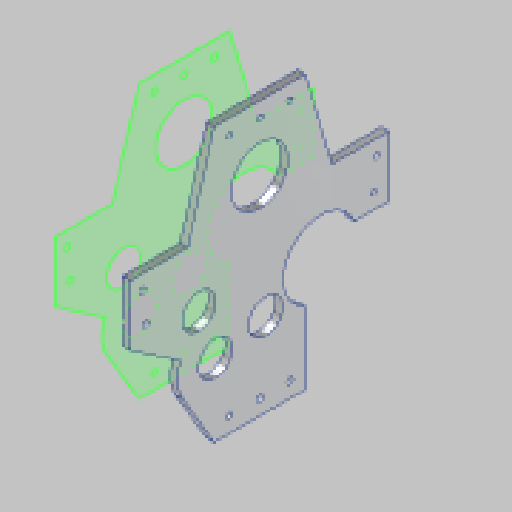
# Autodesk Inventor part: EL2-CGB-003
Saved by Autodesk Inventor 2023.5 (Build 275446000, 446)
## iProperties
Created: 2025-01-19
Part Number: EL2-CGB-003
Material: Aluminum 6061
Document SubType Name: Modeling
Designer: mavericks
Density: 2.7 g/cm^3
Appearance: Aluminum - Flat
Author: mavericks
Autodesk Inventor part; units mm, degrees
ref_plane "YZ Plane" through (0, 0, 0) normal (1, 0, 0) x (0, 1, 0)
ref_plane "XZ Plane" through (0, 0, 0) normal (0, 1, 0) x (-1, 0, 0)
ref_plane "XY Plane" through (0, 0, 0) normal (0, 0, 1) x (1, 0, 0)
sketch "Sketch1" plane through (0, 0, 0) normal (1, 0, 0) x (0, 1, 0)
  line L0 (127, 107.95) -> (-127, 107.95) construction
  line L1 (-127, 107.95) -> (-127, 82.55) construction
  line L2 (-127, 82.55) -> (127, 82.55) construction
  line L3 (127, 82.55) -> (127, 107.95) construction
  line L4 (-44.45, 128.7526) -> (-69.85, 128.7526) construction
  line L5 (-69.85, 128.7526) -> (-69.85, 79.4258) construction
  line L6 (-69.85, 79.4258) -> (-44.45, 79.4258) construction
  line L7 (-44.45, 79.4258) -> (-44.45, 128.7526) construction
  line L8 (69.85, 128.7526) -> (44.45, 128.7526) construction
  line L9 (44.45, 128.7526) -> (44.45, 79.4258) construction
  line L10 (44.45, 79.4258) -> (69.85, 79.4258) construction
  line L11 (69.85, 79.4258) -> (69.85, 128.7526) construction
  line L12 (44.45, 104.0892) -> (-44.45, 104.0892) construction
  line L13 (0, 0) -> (-27.2932, 0) construction
  line L14 (127, -107.95) -> (-127, -107.95) construction
  line L15 (-127, -107.95) -> (-127, -82.55) construction
  line L16 (-127, -82.55) -> (127, -82.55) construction
  line L17 (127, -82.55) -> (127, -107.95) construction
  line L18 (-44.45, -128.7526) -> (-69.85, -128.7526) construction
  line L19 (-69.85, -128.7526) -> (-69.85, -79.4258) construction
  line L20 (-69.85, -79.4258) -> (-44.45, -79.4258) construction
  line L21 (-44.45, -79.4258) -> (-44.45, -128.7526) construction
  line L22 (69.85, -128.7526) -> (44.45, -128.7526) construction
  line L23 (44.45, -128.7526) -> (44.45, -79.4258) construction
  line L24 (44.45, -79.4258) -> (69.85, -79.4258) construction
  line L25 (69.85, -79.4258) -> (69.85, -128.7526) construction
  line L26 (44.45, -104.0892) -> (-44.45, -104.0892) construction
  line L27 (127, 82.55) -> (101.6, 82.55) construction
  line L28 (101.6, 82.55) -> (101.6, -82.55) construction
  line L29 (101.6, -82.55) -> (127, -82.55) construction
  line L30 (127, -82.55) -> (127, 82.55) construction
  line L31 (-127, 82.55) -> (-101.6, 82.55) construction
  line L32 (-101.6, 82.55) -> (-101.6, -82.55) construction
  line L33 (-101.6, -82.55) -> (-127, -82.55) construction
  line L34 (-127, -82.55) -> (-127, 82.55) construction
  point P0 (0, 82.55)
  point P1 (0, 104.0892)
  point P2 (0, -82.55)
  point P3 (0, -104.0892)
  dimension "d0" = 254
  dimension "d1" = 25.4
  dimension "d2" = 82.55
  dimension "d3" = 25.4
  dimension "d4" = 49.3268
  dimension "d6" = 88.9
  dimension "d7" = 3.1242
  dimension "d8" = 25.4
  dimension "d9" = 25.4
  constraints: 70 end point, 16 symmetric about line, 12 parallel, 7 horizontal, 5 perpendicular, 4 midpoint, 2 vertical alignment, 1 horizontal alignment, 1 point on line
  measures "d0" distance of L2.end L1.end
  measures "d1" distance of L1.end L0.end
  measures "d2" vertical distance of L13.start L2.end
  measures "d3" distance of L6.end L5.end
  measures "d4" distance of L5.end L4.end
  measures "d6" distance of L4.start L8.end
  measures "d7" distance from line of L2 L6.end
  measures "d8" distance between parallel lines of L28 L30
  measures "d9" distance between parallel lines of L34 L32
sketch "Sketch2" plane through (0, 0, 0) normal (1, 0, 0) x (0, 1, 0)
  line L0 (-127, 107.95) -> (-127, 82.55) construction
  line L1 (44.45, 104.0892) -> (-44.45, 104.0892) construction
  line L2 (-127, 82.55) -> (127, 82.55) construction
  line L3 (127, 107.95) -> (-127, 107.95) construction
  line L4 (44.45, 79.4258) -> (69.85, 79.4258) construction
  line L5 (127, 82.55) -> (127, 107.95) construction
  line L6 (-69.85, 79.4258) -> (-44.45, 79.4258) construction
  line L7 (-44.45, 79.4258) -> (-44.45, 128.7526) construction
  line L8 (-69.85, 128.7526) -> (-69.85, 79.4258) construction
  line L9 (-44.45, 128.7526) -> (-69.85, 128.7526) construction
  line L10 (101.6, 82.55) -> (101.6, -82.55) construction
  line L11 (127, -82.55) -> (127, 82.55) construction
  line L12 (-127, -82.55) -> (127, -82.55) construction
  line L13 (127, -107.95) -> (-127, -107.95) construction
  line L14 (44.45, -104.0892) -> (-44.45, -104.0892) construction
  line L15 (-127, 82.55) -> (-101.6, 82.55) construction
  line L16 (-101.6, 82.55) -> (-101.6, -82.55) construction
  line L17 (-127, -82.55) -> (-127, 82.55) construction
  line L18 (-69.85, -79.4258) -> (-44.45, -79.4258) construction
  line L19 (-101.6, -82.55) -> (-127, -82.55) construction
  line L20 (-44.45, -79.4258) -> (-44.45, -128.7526) construction
  line L21 (-44.45, -128.7526) -> (-69.85, -128.7526) construction
  line L22 (-69.85, -128.7526) -> (-69.85, -79.4258) construction
  line L23 (-127, -107.95) -> (-127, -82.55) construction
  line L24 (44.45, -79.4258) -> (69.85, -79.4258) construction
  line L25 (44.45, -128.7526) -> (44.45, -79.4258) construction
  line L26 (101.6, -82.55) -> (127, -82.55) construction
  line L27 (69.85, -128.7526) -> (44.45, -128.7526) construction
  line L28 (69.85, -79.4258) -> (69.85, -128.7526) construction
  line L29 (127, -82.55) -> (127, -107.95) construction
  line L30 (69.85, 128.7526) -> (44.45, 128.7526) construction
  line L31 (44.45, 128.7526) -> (44.45, 79.4258) construction
  line L32 (69.85, 79.4258) -> (69.85, 128.7526) construction
  line L33 (127, 82.55) -> (101.6, 82.55) construction
  circle A0 centre (-38.1, -50.8) radius 7.62 construction
  circle A1 centre (-57.15, -5.08) radius 41.91 construction
  circle A2 centre (-57.15, -5.08) radius 11.43 construction
  circle A3 centre (-66.675, 37.0363) radius 31.75 construction
  circle A4 centre (-66.675, 37.0363) radius 15.24 construction
  circle A5 centre (-25.7473, 50.8) radius 27.94 construction
  circle A6 centre (-38.1, -50.8) radius 31.115 construction
  circle A7 centre (-38.1, -50.8) radius 10.16 construction
  circle A8 centre (-57.15, -5.08) radius 14.2875
  circle A9 centre (-66.675, 37.0363) radius 14.2875
  circle A10 centre (-25.7473, 50.8) radius 14.2875
  circle A11 centre (-25.7473, 50.8) radius 20.6375 construction
  circle A12 centre (-66.675, 37.0363) radius 20.6375 construction
  circle A13 centre (-57.15, -5.08) radius 20.6375 construction
  circle A14 centre (-38.1, -50.8) radius 17.4625 construction
  circle A15 centre (-38.1, -50.8) radius 25.4 construction
  line L34 (-41.275, -131.9276) -> (-41.275, -76.2508) construction
  line L35 (-41.275, -76.2508) -> (-73.025, -76.2508) construction
  line L36 (-73.025, -76.2508) -> (-73.025, -131.9276) construction
  line L37 (-73.025, -131.9276) -> (-41.275, -131.9276) construction
  line L38 (-127, -38.1) -> (-127, 38.1)
  line L39 (-127, 38.1) -> (-41.275, 38.1) construction
  line L40 (-41.275, 38.1) -> (-41.275, 104.0892) construction
  circle A16 centre (-38.1, -50.8) radius 31.115
  circle A17 centre (86.4755, 0) radius 23.8125
  circle A18 centre (86.4755, 0) radius 33.3375 construction
  line L41 (37.9487, 60.325) -> (127, 38.1)
  line L42 (127, 38.1) -> (127, -38.1)
  line L43 (127, -38.1) -> (37.9487, -60.325)
  line L44 (37.9487, -60.325) -> (37.9487, -107.95)
  line L45 (37.9487, -107.95) -> (-12.7, -107.95)
  line L46 (37.9487, 60.325) -> (37.9487, 107.95)
  line L47 (37.9487, 107.95) -> (-12.7, 107.95)
  arc A19 (-23.4758, 68.844) -> (-37.8063, 37.1865) centre (-25.7473, 50.8) ccw construction
  arc A20 (50.2903, -40.85) -> (93.2916, 54.1446) centre (86.4755, 0) ccw construction
  line L48 (-12.7, 107.95) -> (-41.275, 56.0863)
  line L49 (-82.9044, 64.325) -> (-127, 38.1)
  arc A21 (-41.275, 56.0863) -> (-82.9044, 64.325) centre (-66.675, 37.0363) ccw
  line L50 (-66.5052, -38.1) -> (-127, -38.1)
  line L51 (-12.7, -68.7717) -> (-12.7, -107.95)
  line L52 (-23.4758, 68.844) -> (93.2916, 54.1446) construction
  line L53 (-37.8063, 37.1865) -> (50.2903, -40.85) construction
  point P0 (25.2487, 98.0186)
  point P1 (0, 95.25)
  point P2 (25.2487, -98.0186)
  point P3 (0, -95.25)
  point P4 (-25.4, -95.25)
  point P5 (-25.4, 95.25)
  point P6 (127, -95.25)
  point P7 (127, 95.25)
  point P8 (0, -82.55)
  point P9 (-114.3, 25.4)
  point P10 (-114.3, 0)
  point P11 (-114.3, -25.4)
  point P12 (-101.6, 0)
  point P13 (-114.3, 82.55)
  point P14 (-38.1, -25.4)
  point P15 (-38.1, -33.3375)
  point P16 (-60.097, -38.1)
  point P17 (-53.223, -42.0688)
  point P18 (-60.097, -63.5)
  point P19 (-53.223, -59.5312)
  point P20 (-38.1, -76.2)
  point P21 (-38.1, -68.2625)
  point P22 (-16.103, -63.5)
  point P23 (-22.977, -59.5313)
  point P24 (-16.103, -38.1)
  point P25 (-22.977, -42.0688)
  point P26 (44.45, 104.0892)
  point P27 (-41.275, -81.7526)
  point P28 (-127, 0)
  point P29 (-127, 0)
  point P30 (101.6, 0)
  point P31 (114.3, 25.4)
  point P32 (114.3, 0)
  point P33 (114.3, -25.4)
  point P34 (114.3, 82.55)
  point P35 (127, 0)
  dimension "d33" = 34.925
  dimension "d34" = 50.8
  dimension "d10" = 15.24
  dimension "d11" = 83.82
  dimension "d12" = 22.86
  dimension "d13" = 63.5
  dimension "d14" = 30.48
  dimension "d15" = 55.88
  dimension "d16" = 62.23
  dimension "d19" = 63.5
  dimension "d23" = 20.32
  dimension "d24" = 28.575
  dimension "d26" = 25.4
  dimension "d27" = 25.4
  dimension "d28" = 25.4
  dimension "d29" = 25.4
  dimension "d30" = 6.35
  dimension "d31" = 6.35
  dimension "d32" = 6.35
  dimension "d37" = 360
  dimension "d41" = 3.175
  dimension "d42" = 76.2
  dimension "d60" = 101.7513
  dimension "d63" = 31.75
  dimension "d64" = 44.45
  dimension "d66" = 34.925
  dimension "d67" = 31.75
  dimension "d68" = 47.625
  dimension "d70" = 9.525
  dimension "d71" = 47.625
  dimension "d73" = 123.1853
  dimension "d74" = 12.7
  dimension "d75" = 36.3728
  dimension "d76" = 109.1438
  dimension "d78" = 9.9314
  dimension "d79" = 9.9314
  dimension "d137" = 12.7
  dimension "d149" = 204.1689
  dimension "d151" = 46.2281
  dimension "d152" = 117.689
  constraints: 41 end point, 20 centre point, 18 vertical alignment, 14 coincident, 12 point on circle, 11 horizontal alignment, 11 midpoint, 10 point on line, 8 tangent, 3 perpendicular, 2 collinear, 2 equal radius, 2 horizontal, 1 vertical, 20 other
  measures "d10" diameter of A0
  measures "d11" diameter of A1
  measures "d12" diameter of A2
  measures "d13" diameter of A3
  measures "d14" diameter of A4
  measures "d15" diameter of A5
  measures "d16" diameter of A6
  measures "d19" distance from line of L16 A0.centre
  measures "d23" diameter of A7
  measures "d24" diameter of A8
  measures "d26" distance of point (-25.4, 95.25) point (0, 95.25)
  measures "d27" distance of point (25.249, 98.019) point (0, 95.25)
  measures "d28" distance of point (-114.3, 0) point (-114.3, 25.4)
  measures "d29" distance of point (-114.3, 0) point (-114.3, -25.4)
  measures "d30" radial gap between concentric circles of A10 A11
  measures "d31" radial gap between concentric circles of A9 A12
  measures "d32" radial gap between concentric circles of A8 A13
  measures "d41" distance between parallel lines of L20 L34
  measures "d42" distance of L38.start L38.end
  measures "d60" distance from line of L5 point (25.249, 98.019)
  measures "d63" distance from line of L12 A0.centre
  measures "d64" distance from line of L16 A1.centre
  measures "d66" distance from line of L16 A3.centre
  measures "d67" distance from line of L2 A5.centre
  measures "d68" diameter of A17
  measures "d70" radial gap between concentric circles of A17 A18
  measures "d71" distance of L41.start L46.end
  measures "d73" distance of A17.centre A5.centre
  measures "d74" horizontal distance of point (25.249, 98.019) L46.end
  measures "d75" diameter of A19
  measures "d76" diameter of A20
  measures "d78" distance from line of point (25.249, 98.019) L3
  measures "d79" distance from line of L13 point (25.249, -98.019)
  measures "d137" distance from line of L51 point (0, -95.25)
  measures "d152" distance of L52.start L52.end
extrude "Extrusion1" add sketch "Sketch2" along normal blind 6.35 contours L38 L49 A21 L48 L47 L46 L41 L42 L43 L44 L45 L51 A16 L50
hole "Mount Holes" at (0, -101.6, 82.55) at (0, -127, 107.95) at (0, -69.85, 79.4258) at (0, -44.45, -79.4258) at (0, 44.45, -79.4258) at (0, 69.85, -79.4258) at (0, 44.45, -128.7526) at (0, 44.45, 128.7526) at (0, 25.2487, 98.0186) at (0, 0, 95.25) at (0, 25.2487, -98.0186) at (0, 0, -95.25) at (0, -25.4, -95.25) at (0, -25.4, 95.25) at (0, -114.3, 25.4) at (0, -114.3, 0) at (0, -114.3, -25.4) at (0, 114.3, 25.4) at (0, 114.3, 0) at (0, 114.3, -25.4) direction (1, 0, 0) diameter 5.1054 end through all clearance for "Flat Head Machine Screw (82)" size "#10" standard "Ansi Unified Screw Threads"
sketch "Sketch5" plane through (6.35, 0, 0) normal (1, 0, 0) x (0, 0, -1)
  circle A0 centre (25.4, -114.3) radius 2.5527 projected
  circle A1 centre (-25.4, -114.3) radius 2.5527 projected
  circle A2 centre (98.0186, 25.2487) radius 2.5527 projected
  circle A3 centre (-98.0186, 25.2487) radius 2.5527 projected
  circle A4 centre (-95.25, 0) radius 2.5527 projected
  circle A5 centre (95.25, 0) radius 2.5527 projected
  circle A6 centre (0, -114.3) radius 2.5527 projected
  circle A7 centre (-25.4, 114.3) radius 2.5527 projected
  circle A8 centre (25.4, 114.3) radius 2.5527 projected
  circle A9 centre (5.08, -57.15) radius 14.2875 projected
  circle A10 centre (-37.0363, -66.675) radius 14.2875 projected
  circle A11 centre (-50.8, -25.7473) radius 14.2875 projected
  circle A12 centre (0, 86.4755) radius 23.8125 projected
  line L0 (38.1, -127) -> (-38.1, -127) projected
  line L1 (-38.1, -127) -> (-64.325, -82.9044) projected
  arc A13 (-56.0863, -41.275) -> (-64.325, -82.9044) centre (-37.0363, -66.675) ccw projected
  line L2 (-56.0863, -41.275) -> (-107.95, -12.7) projected
  line L3 (-107.95, -12.7) -> (-107.95, 37.9487) projected
  line L4 (-107.95, 37.9487) -> (-60.325, 37.9487) projected
  line L5 (-60.325, 37.9487) -> (-38.1, 127) projected
  line L6 (-38.1, 127) -> (38.1, 127) projected
  line L7 (38.1, 127) -> (60.325, 37.9487) projected
  line L8 (60.325, 37.9487) -> (107.95, 37.9487) projected
  line L9 (107.95, 37.9487) -> (107.95, -12.7) projected
  line L10 (38.1, -66.5052) -> (38.1, -127) projected
  line L11 (54.5703, 34.783) -> (33.14, 120.65) construction
  line L12 (33.14, 120.65) -> (-33.14, 120.65) construction
  line L13 (-33.14, 120.65) -> (-55.365, 31.5987) construction
  line L14 (-55.365, 31.5987) -> (-101.6, 31.5987) construction
  line L15 (-101.6, 31.5987) -> (-101.6, -8.9486) construction
  line L16 (-101.6, -8.9486) -> (-42.0284, -41.7704) construction
  arc A14 (-42.0284, -41.7704) -> (-58.8673, -79.6585) centre (-37.0363, -66.675) ccw construction
  line L17 (-58.8673, -79.6585) -> (-34.4884, -120.65) construction
  line L18 (-34.4884, -120.65) -> (31.75, -120.65) construction
  line L19 (31.75, -120.65) -> (31.75, -59.587) construction
  arc A15 (89.8157, -28.4708) -> (31.75, -59.587) centre (50.8, -25.4) ccw construction
  line L20 (89.8157, -28.4708) -> (104.7843, -25.6998) construction
  line L21 (104.7843, -25.6998) -> (104.7843, 34.783) construction
  line L22 (104.7843, 34.783) -> (54.5703, 34.783) construction
  circle A16 centre (0, 86.4755) radius 33.3375 construction
  circle A17 centre (5.08, -57.15) radius 20.6375 construction
  circle A18 centre (-37.0363, -66.675) radius 20.6375 construction
  circle A19 centre (-50.8, -25.7473) radius 20.6375 construction
  circle A20 centre (-95.25, 0) radius 8.9027 construction
  circle A21 centre (-98.0186, 25.2487) radius 8.9027 construction
  circle A22 centre (-95.25, -25.4) radius 8.9027 construction
  circle A23 centre (95.25, -25.4) radius 8.9027 construction
  circle A24 centre (95.25, 0) radius 8.9027 construction
  circle A25 centre (98.0186, 25.2487) radius 8.9027 construction
  circle A26 centre (-25.4, -114.3) radius 8.9027 construction
  circle A27 centre (0, -114.3) radius 8.9027 construction
  circle A28 centre (25.4, -114.3) radius 8.9027 construction
  line L23 (107.95, -12.7) -> (68.7717, -12.7) projected
  arc A29 (68.7717, -12.7) -> (38.1, -66.5052) centre (50.8, -38.1) ccw projected
  circle A30 centre (0, 114.3) radius 2.5527 projected
  point P0 (0, 0)
  point P1 (23.4598, 103.2589)
  point P2 (18.3925, 114.3)
  dimension "d123" = 6.35
  dimension "d124" = 9.525
  dimension "d125" = 6.35
  dimension "d126" = 6.35
  dimension "d127" = 6.35
  dimension "d128" = 6.35
  dimension "d129" = 6.35
  dimension "d132" = 6.35
  dimension "d133" = 6.35
  dimension "d134" = 6.35
  dimension "d135" = 6.35
  dimension "d136" = 6.35
  constraints: 24 end point, 15 centre point, 4 point on circle, 10 other
  measures "d123" distance between parallel lines of L7 L11
  measures "d124" radial gap between concentric circles of A12 A16
  measures "d125" radial gap between concentric circles of A9 A17
  measures "d126" radial gap between concentric circles of A10 A18
  measures "d127" radial gap between concentric circles of A11 A19
  measures "d128" radial gap between concentric circles of A4 A20
  measures "d129" radial gap between concentric circles of A3 A21
  measures "d132" radial gap between concentric circles of A5 A24
  measures "d133" radial gap between concentric circles of A2 A25
  measures "d134" radial gap between concentric circles of A1 A26
  measures "d135" radial gap between concentric circles of A6 A27
  measures "d136" radial gap between concentric circles of A0 A28
sketch "Sketch6" plane through (6.35, 0, 0) normal (1, 0, 0) x (0, 0, -1)
  circle A0 centre (0, 101.6) radius 2.5527 projected
  circle A1 centre (25.4, -101.6) radius 2.5527 projected
  circle A2 centre (-25.4, -101.6) radius 2.5527 projected
  circle A3 centre (98.0186, 25.2487) radius 2.5527 projected
  circle A4 centre (-98.0186, 25.2487) radius 2.5527 projected
  circle A5 centre (-95.25, 0) radius 2.5527 projected
  circle A6 centre (95.25, 0) radius 2.5527 projected
  circle A7 centre (0, -101.6) radius 2.5527 projected
  circle A8 centre (-25.4, 101.6) radius 2.5527 projected
  circle A9 centre (25.4, 101.6) radius 2.5527 projected
  circle A10 centre (5.08, -44.45) radius 14.2875 projected
  circle A11 centre (-37.0363, -53.975) radius 14.2875 projected
  circle A12 centre (-50.8, -13.0473) radius 14.2875 projected
  circle A13 centre (0, 59.9086) radius 23.8125 projected
  line L0 (38.1, -114.3) -> (-38.1, -114.3) projected
  line L1 (-38.1, -114.3) -> (-64.325, -70.2044) projected
  arc A14 (-66.1357, -41.275) -> (-64.325, -70.2044) centre (-37.0363, -53.975) ccw projected
  line L2 (-66.1357, -41.275) -> (-107.95, -12.7) projected
  line L3 (-107.95, -12.7) -> (-107.95, 37.9487) projected
  line L4 (-107.95, 37.9487) -> (-60.325, 37.9487) projected
  line L5 (-60.325, 37.9487) -> (-38.1, 114.3) projected
  line L6 (-38.1, 114.3) -> (38.1, 114.3) projected
  line L7 (38.1, 114.3) -> (60.325, 37.9487) projected
  line L8 (60.325, 37.9487) -> (107.95, 37.9487) projected
  line L9 (107.95, 37.9487) -> (107.95, -12.7) projected
  line L10 (107.95, -12.7) -> (79.2052, -12.7) projected
  arc A15 (79.2052, -12.7) -> (38.1, -53.8052) centre (50.8, -25.4) ccw projected
  line L11 (38.1, -53.8052) -> (38.1, -114.3) projected
  line L12 (-33.3349, 107.95) -> (-55.5599, 31.5987) construction
  line L13 (-55.5599, 31.5987) -> (-101.6, 31.5987) construction
  line L14 (-101.6, 31.5987) -> (-101.6, -9.3483) construction
  line L15 (-101.6, -9.3483) -> (-57.7691, -39.3014) construction
  arc A16 (-57.7691, -39.3014) -> (-58.8673, -66.9585) centre (-37.0363, -53.975) ccw construction
  line L16 (-58.8673, -66.9585) -> (-34.4884, -107.95) construction
  line L17 (-34.4884, -107.95) -> (31.75, -107.95) construction
  line L18 (31.75, -107.95) -> (31.75, -57.6602) construction
  arc A17 (83.0602, -6.35) -> (31.75, -57.6602) centre (50.8, -25.4) ccw construction
  line L19 (83.0602, -6.35) -> (101.6, -6.35) construction
  line L20 (101.6, -6.35) -> (101.6, 31.5987) construction
  line L21 (101.6, 31.5987) -> (55.5599, 31.5987) construction
  line L22 (55.5599, 31.5987) -> (33.3349, 107.95) construction
  line L23 (33.3349, 107.95) -> (-33.3349, 107.95) construction
  circle A18 centre (-50.8, -13.0473) radius 20.6375 construction
  circle A19 centre (-37.0363, -53.975) radius 20.6375 construction
  circle A20 centre (5.08, -44.45) radius 20.6375 construction
  circle A21 centre (-98.0186, 25.2487) radius 8.9027 construction
  circle A22 centre (-95.25, 0) radius 8.9027 construction
  circle A23 centre (-25.4, -101.6) radius 8.9027 construction
  circle A24 centre (0, -101.6) radius 8.9027 construction
  circle A25 centre (25.4, -101.6) radius 8.9027 construction
  circle A26 centre (95.25, 0) radius 8.9027 construction
  circle A27 centre (98.0186, 25.2487) radius 8.9027 construction
  circle A28 centre (25.4, 101.6) radius 8.9027 construction
  circle A29 centre (0, 101.6) radius 8.9027 construction
  circle A30 centre (-25.4, 101.6) radius 8.9027 construction
  circle A31 centre (0, 59.9086) radius 33.3375 construction
  line L24 (-50.8, -13.0473) -> (0, 59.9086) construction
  line L25 (0, 59.9086) -> (50.8, -25.4) construction
  line L26 (-48.0336, -14.6307) -> (-0.2084, 54.0531) construction
  line L27 (-0.2084, 54.0531) -> (48.072, -27.0245) construction
  line L28 (-53.3988, -11.2234) -> (0.2084, 65.7642) construction
  line L29 (0.2084, 65.7642) -> (53.528, -23.7755) construction
  line L30 (-48.1662, 56.9987) -> (-33.2103, 56.9987) construction
  line L31 (33.2103, 56.9987) -> (48.1662, 56.9987) construction
  line L32 (-86.7077, -2.5074) -> (-70.6021, -7.2349) construction
  line L33 (-16.3578, 30.8602) -> (-36.542, 1.873)
  line L34 (14.2513, 29.7708) -> (28.9724, 5.0497)
  line L35 (-91.7788, 31.5987) -> (-55.5599, 31.5987)
  line L36 (-55.5599, 31.5987) -> (-48.1662, 56.9987)
  line L37 (-48.1662, 56.9987) -> (-33.2103, 56.9987)
  line L38 (33.2103, 56.9987) -> (48.1662, 56.9987)
  line L39 (48.1662, 56.9987) -> (55.5599, 31.5987)
  line L40 (55.5599, 31.5987) -> (91.7788, 31.5987)
  line L41 (-86.7077, -2.5074) -> (-70.6021, -7.2349)
  line L42 (-101.6, 17.0981) -> (-101.6, 6.2398)
  line L43 (-44.2218, -32.6083) -> (-43.6146, -34.414)
  line L44 (-16.9072, -49.4226) -> (-15.0491, -49.0024)
  circle A32 centre (-98.0186, 25.2487) radius 2.5527 projected
  arc A33 (-101.6, 17.0981) -> (-91.7788, 31.5987) centre (-98.0186, 25.2487) ccw
  arc A34 (-86.7077, -2.5074) -> (-101.6, 6.2398) centre (-95.25, 0) ccw
  arc A35 (-41.7531, 5.5015) -> (-70.6021, -7.2349) centre (-50.8, -13.0473) ccw
  arc A36 (-33.2103, 56.9987) -> (-21.569, 34.4888) centre (0, 59.9086) ccw
  arc A37 (19.7072, 33.0197) -> (33.2103, 56.9987) centre (0, 59.9086) ccw
  arc A38 (28.9724, 5.0497) -> (13.3352, -25.5355) centre (50.8, -25.4) ccw
  arc A39 (13.3352, -25.5355) -> (-15.0491, -49.0024) centre (5.08, -44.45) ccw
  arc A40 (-16.9072, -49.4226) -> (-43.6146, -34.414) centre (-37.0363, -53.975) ccw
  arc A41 (-44.2218, -32.6083) -> (-36.542, 1.873) centre (-50.8, -13.0473) ccw
  arc A42 (83.0602, -6.35) -> (34.4283, 8.2986) centre (50.8, -25.4) ccw
  circle A43 centre (95.25, 0) radius 2.5527 projected
  arc A44 (101.6, 6.2398) -> (89.0102, -6.35) centre (95.25, 0) ccw
  circle A45 centre (98.0186, 25.2487) radius 2.5527 projected
  arc A46 (91.7788, 31.5987) -> (101.6, 17.0981) centre (98.0186, 25.2487) ccw
  arc A47 (-16.3578, 30.8602) -> (14.2513, 29.7708) centre (0, 59.9086) ccw
  line L45 (101.6, 6.2398) -> (101.6, 17.0981)
  line L46 (89.0102, -6.35) -> (83.0602, -6.35)
  line L47 (-58.8673, -66.9585) -> (-54.774, -64.5241)
  line L48 (-32.484, -74.1041) -> (9.6324, -64.5791)
  arc A48 (-54.774, -64.5241) -> (-32.484, -74.1041) centre (-37.0363, -53.975) ccw
  arc A49 (9.6324, -64.5791) -> (24.3233, -51.9068) centre (5.08, -44.45) ccw
  arc A50 (24.3233, -51.9068) -> (31.75, -57.6602) centre (50.8, -25.4) ccw
  circle A51 centre (25.4, -114.3) radius 2.5527 projected
  arc A52 (31.75, -95.3602) -> (19.1602, -107.95) centre (25.4, -101.6) ccw
  circle A53 centre (0, -114.3) radius 2.5527 projected
  arc A54 (6.2398, -107.95) -> (-6.2398, -107.95) centre (0, -101.6) ccw
  circle A55 centre (-25.4, -114.3) radius 2.5527 projected
  arc A56 (-19.1602, -107.95) -> (-29.9507, -93.9483) centre (-25.4, -101.6) ccw
  line L49 (-39.4542, -99.6003) -> (-29.9507, -93.9483)
  line L50 (-19.1602, -107.95) -> (-6.2398, -107.95)
  line L51 (6.2398, -107.95) -> (19.1602, -107.95)
  line L52 (-39.4542, -99.6003) -> (-58.8673, -66.9585)
  line L53 (31.75, -95.3602) -> (31.75, -57.6602)
  line L54 (-21.569, 34.4888) -> (-41.7531, 5.5015)
  line L55 (19.7072, 33.0197) -> (34.4283, 8.2986)
  point P0 (0, 0)
  dimension "d138" = 6.35
  dimension "d139" = 6.35
  dimension "d140" = 6.35
  dimension "d141" = 9.525
  dimension "d142" = 3.175
  dimension "d143" = 3.175
  dimension "d144" = 25.4
  constraints: 90 end point, 79 point on circle, 34 centre point, 24 point on line, 17 coincident, 11 collinear, 9 equal radius, 8 line through centre, 3 concentric, 3 vertical alignment, 2 perpendicular, 2 tangent, 1 horizontal, 21 other
  measures "d138" distance between parallel lines of L5 L12
  measures "d139" radial gap between concentric circles of A12 A18
  measures "d140" radial gap between concentric circles of A4 A21
  measures "d141" radial gap between concentric circles of A13 A31
  measures "d142" distance between parallel lines of L24 L26
  measures "d143" distance between parallel lines of L24 L28
  measures "d144" distance between parallel lines of L13 L30
body "Solid1"
